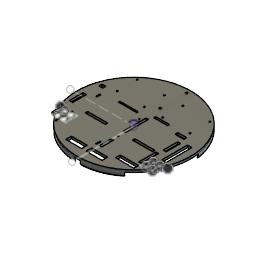
base (Autodesk Fusion 360 design; units mm, degrees)
part number: 2026-05-09-09-08-22-540
Autodesk Fusion 360 part; units mm, degrees
note: some values were not read from the file. Chosen so that the rebuilt part matches the saved one: which face or edge a step refers to. Set by a fixed rule: which sketch regions a step uses.
(part 1 of 2)
sketch "Sketch1" plane through (0, 0, 0) normal (0, 1, 0) x (1, 0, 0)
  circle A0 centre (0, 0) radius 125
  dimension "d1" = 250
  constraint coincident A0.centre origin
  measures "d1" diameter of A0
extrude "Extrude1" add sketch "Sketch1" along normal blind 5 makes body 1
sketch "Sketch3" plane through (0, 0, 0) normal (0, -1, 0) x (1, 0, 0)
  circle A0 centre (0, 0) radius 125
  line L0 (10, -45) -> (-10, -45)
  line L1 (-10, -45) -> (-10, -205)
  line L2 (-10, -205) -> (10, -205)
  line L3 (10, -205) -> (10, -45)
  line L4 (10, -45) -> (-10, -205) construction
  line L5 (-10, -45) -> (10, -205) construction
  point P0 (0, -125)
  dimension "d6" = 20
  dimension "d7" = 160
  constraint horizontal L0
  constraint perpendicular L0 L1
  constraint parallel L0 L2
  constraint parallel L1 L3
  constraint coincident L4 P0
  constraint coincident L5 P0
  constraint coincident A0 P0
  measures "d6" distance of L1.end L2.end
  measures "d7" distance of L0.end L1.end
extrude "Extrude2" add sketch "Sketch3" along normal blind 14 contours A0 L0 L1 L3 picked at (1.1122, -71.6518) bodies 1
sketch "Sketch4" plane through (0, -14, 0) normal (0, -1, 0) x (1, 0, 0)
  arc A0 (-10, -124.5994) -> (10, -124.5994) centre (0, 0) ccw
  line L0 (10, -124.5994) -> (10, -45)
  line L1 (10, -45) -> (-10, -45)
  line L2 (-10, -45) -> (-10, -124.5994)
  circle A1 centre (0, -116) radius 2.45
  circle A2 centre (0, -58) radius 2.45
  dimension "d10" = 4.9
  dimension "d11" = 4.9
  dimension "d13" = 58
  measures "d10" diameter of A1
  measures "d11" diameter of A2
  measures "d13" vertical distance of A1.centre A2.centre
extrude "Extrude3" cut sketch "Sketch4" against normal blind 19 contours A1 | A2 bodies 1
sketch "Sketch5" plane through (0, 0, 0) normal (0, -1, 0) x (1, 0, 0)
  line L0 (10, -45) -> (10, -124.5994)
  arc A0 (10, -124.5994) -> (-10, -124.5994) centre (0, 0) ccw
  line L1 (-10, -124.5994) -> (-10, -45)
  line L2 (-10, -45) -> (10, -45)
  line L3 (90.95, 48) -> (104.95, 48)
  line L4 (104.95, 48) -> (104.95, 64)
  line L5 (104.95, 64) -> (90.95, 64)
  line L6 (90.95, 64) -> (90.95, 48)
  line L7 (112.5, 43.0811) -> (82.5, 43.0811)
  line L8 (82.5, 43.0811) -> (82.5, 68.0811)
  line L9 (82.5, 68.0811) -> (112.5, 68.0811)
  line L10 (112.5, 68.0811) -> (112.5, 43.0811)
  circle A1 centre (104.95, 64) radius 1.5
  circle A2 centre (90.95, 64) radius 1.5
  circle A3 centre (90.95, 48) radius 1.5
  circle A4 centre (104.95, 48) radius 1.5
  line L11 (0, 0) -> (0, 135.933)
  circle A5 centre (-104.95, 64) radius 1.5
  line L12 (-90.95, 64) -> (-90.95, 48)
  line L13 (-104.95, 48) -> (-104.95, 64)
  circle A6 centre (-90.95, 64) radius 1.5
  circle A7 centre (-104.95, 48) radius 1.5
  line L14 (-112.5, 43.0811) -> (-82.5, 43.0811)
  line L15 (-104.95, 64) -> (-90.95, 64)
  line L16 (-112.5, 68.0811) -> (-112.5, 43.0811)
  line L17 (-90.95, 48) -> (-104.95, 48)
  line L18 (-82.5, 43.0811) -> (-82.5, 68.0811)
  circle A8 centre (-90.95, 48) radius 1.5
  line L19 (-82.5, 68.0811) -> (-112.5, 68.0811)
  line L20 (-112.5, 43.0811) -> (-117.3415, 43.0811)
  line L21 (112.5, 43.0811) -> (117.3415, 43.0811)
  line L22 (-82.5, 55.5811) -> (-112.5, 55.5811) construction
  line L23 (-97.5, 43.0811) -> (-97.5, 55.5811) construction
  line L24 (0, 0) -> (-140, 0) construction
  dimension "d22" = 14
  dimension "d23" = 16
  dimension "d24" = 93
  dimension "d29" = 30
  dimension "d30" = 25
  dimension "d32" = 7.55
  dimension "d33" = 4.0811
  dimension "d34" = 3
  dimension "d35" = 3
  dimension "d36" = 3
  dimension "d37" = 3
  dimension "d145" = 225
  constraint horizontal L3
  constraint vertical L4
  constraint horizontal L5
  constraint vertical L6
  constraint horizontal L7
  constraint vertical L8
  constraint horizontal L9
  constraint vertical L10
  constraint coincident L4.end L5.start
  constraint coincident L5.end L6.start
  constraint coincident L3.start L6.end
  constraint coincident L3.end L4.start
  constraint coincident A0.centre L11.start
  constraint vertical L11
  constraint symmetric L3.start L11 L12.end
  constraint symmetric L3.end L11 L13.start
  constraint symmetric L4.end L11 A5.centre
  constraint symmetric L5.end L11 L12.start
  constraint symmetric L7.start L11 L14.start
  constraint symmetric L7.end L11 L14.end
  constraint symmetric L8.end L11 L18.end
  constraint symmetric L9.end L11 L16.start
  constraint symmetric A1 L11 A5
  constraint symmetric A2 L11 A6
  constraint symmetric A3 L11 A8
  constraint symmetric A4 L11 A7
  constraint coincident A0 L20.end
  constraint perpendicular L16 L20
  constraint coincident A0 L21.end
  constraint perpendicular L10 L21
  constraint midpoint L18 L22.start
  constraint midpoint L16 L22.end
  constraint midpoint L14 L23.start
  constraint midpoint L22 L23.end
  constraint perpendicular L11 L24
  measures "d22" distance of L3.start L3.end
  measures "d23" distance of L3.start L5.end
  measures "d24" distance of L2 L3
  measures "d29" distance of L7.start L7.end
  measures "d30" distance of L7.start L9.end
  measures "d32" distance of L4 L10
  measures "d33" distance of L5 L9
  measures "d34" diameter of A1
  measures "d35" diameter of A2
  measures "d36" diameter of A3
  measures "d37" diameter of A4
  measures "d145" distance of L10 L16
extrude "Extrude4" add sketch "Sketch5" against normal blind 5 contours A0 L9 L10 | A0 L16 L19 bodies 1
extrude "Extrude5" cut sketch "Sketch5" against normal blind 5 contours L3 L6 A3 | L3 L6 A3 | L3 L4 A4 | L3 L4 A4 | L5 L6 A2 | L5 L6 A2 | L4 L5 A1 | L4 L5 A1 | A5 L13 L15 | A5 L13 L15 | L12 A6 L15 | L12 A6 L15 | L13 A7 L17 | L13 A7 L17 | L12 L17 A8 | L12 L17 A8 bodies 1
sketch "Sketch6" plane through (0, 5, 0) normal (0, 1, 0) x (-1, 0, 0)
  line L0 (112.5, 54.4862) -> (112.5, 68.0811)
  line L1 (112.5, 68.0811) -> (104.833, 68.0811)
  arc A0 (104.833, 68.0811) -> (-104.833, 68.0811) centre (0, 0) ccw
  line L2 (-104.833, 68.0811) -> (-112.5, 68.0811)
  line L3 (-112.5, 68.0811) -> (-112.5, 54.4862)
  circle A1 centre (0, -58) radius 2.45
  circle A2 centre (0, -116) radius 2.45
  circle A3 centre (104.95, 48) radius 1.5
  circle A4 centre (90.95, 64) radius 1.5
  circle A5 centre (90.95, 48) radius 1.5
  circle A6 centre (-90.95, 64) radius 1.5
  circle A7 centre (-90.95, 48) radius 1.5
  circle A8 centre (-104.95, 48) radius 1.5
  circle A9 centre (0, -58) radius 5
  circle A10 centre (0, -116) radius 5
  line L4 (-97.9276, 40.2238) -> (-97.9276, 63.5811)
  circle A11 centre (-105.0292, 44.701) radius 1.5
  circle A12 centre (-90.9905, 60.7002) radius 1.5
  circle A13 centre (-90.8662, 44.7011) radius 1.5
  circle A14 centre (-104.8647, 60.7002) radius 1.5
  circle A15 centre (-104.989, 44.7011) radius 1.5
  line L5 (0, 0) -> (0, 94)
  circle A16 centre (105.0292, 44.701) radius 1.5
  circle A17 centre (90.8662, 44.7011) radius 1.5
  circle A18 centre (104.8647, 60.7002) radius 1.5
  circle A19 centre (90.8944, 60.7176) radius 1.5
  arc A20 (-112.5, 54.4862) -> (112.5, 54.4862) centre (0, 0) ccw
  circle A21 centre (104.95, 64) radius 1.5
  circle A22 centre (-104.95, 64) radius 1.5
  circle A23 centre (90.9999, 67.3221) radius 1.5
  point P0 (-104.95, 48)
  point P1 (-115.3176, 44.7)
  point P2 (-104.95, 64)
  point P3 (-90.95, 48)
  point P4 (-90.95, 64)
  dimension "d42" = 10
  dimension "d45" = 3
  dimension "d46" = 3.3
  dimension "d49" = 3
  dimension "d50" = 3
  dimension "d51" = 3.3
  dimension "d52" = 3.3
  constraint concentric A1 A9
  constraint concentric A2 A10
  constraint vertical L4
  constraint symmetric L4 A12 A14
  constraint symmetric L4 A13 A15
  constraint coincident A0.centre L5.start
  constraint vertical L5
  constraint symmetric A11 L5 A16
  constraint symmetric A13 L5 A17
  constraint symmetric A14 L5 A18
  measures "d42" diameter of A9
  measures "d45" diameter of A11
  measures "d46" distance of A11.centre P0
  measures "d49" diameter of A12
  measures "d50" diameter of A13
  measures "d51" distance of A13.centre P3
  measures "d52" distance of A12.centre P4
extrude "Extrude7" cut sketch "Sketch6" against normal blind 5 contours A11 A15 | A11 A15 | A12 | A13 | A14 | A16 | A17 | A18 | A19 | A21 | A23 bodies 1
sketch "Sketch7" plane through (0, 0, 0) normal (0, -1, 0) x (1, 0, 0)
  circle A0 centre (104.95, 48) radius 1.5
  arc A1 (10, -124.5994) -> (112.5, 54.4862) centre (0, 0) ccw
  line L0 (-10, -124.5994) -> (-10, -45)
  line L1 (-10, -45) -> (10, -45)
  line L2 (10, -45) -> (10, -124.5994)
  line L3 (112.5, 54.4862) -> (112.5, 68.0811)
  line L4 (112.5, 68.0811) -> (104.833, 68.0811)
  arc A2 (104.833, 68.0811) -> (-104.833, 68.0811) centre (0, 0) ccw
  line L5 (-104.833, 68.0811) -> (-112.5, 68.0811)
  line L6 (-112.5, 68.0811) -> (-112.5, 54.4862)
  circle A3 centre (-90.95, 64) radius 1.5
  circle A4 centre (-90.95, 48) radius 1.5
  circle A5 centre (90.95, 64) radius 1.5
  circle A6 centre (90.95, 48) radius 1.5
  circle A7 centre (-104.95, 48) radius 1.5
  line L7 (0.0614, -38.5696) -> (0.0614, 91.4304)
  line L8 (-72.4386, -5) -> (-69.4386, -5)
  line L9 (-69.4386, -5) -> (-69.4386, -10)
  line L10 (-69.4386, -10) -> (-72.4386, -10)
  line L11 (-72.4386, -10) -> (-72.4386, -5)
  line L12 (72.5614, -5) -> (69.5614, -5)
  line L13 (72.5614, -10) -> (72.5614, -5)
  line L14 (69.5614, -10) -> (72.5614, -10)
  line L15 (69.5614, -5) -> (69.5614, -10)
  line L16 (30, 28) -> (-30, 28)
  line L17 (-30, 28) -> (-30, 25)
  line L18 (-30, 25) -> (30, 25)
  line L19 (30, 25) -> (30, 28)
  arc A8 (-112.5, 54.4862) -> (-10, -124.5994) centre (0, 0) ccw
  circle A9 centre (104.95, 64) radius 1.5
  circle A10 centre (-104.95, 64) radius 1.5
  circle A11 centre (-90.9999, 67.3221) radius 1.5
  circle A12 centre (-105, 52) radius 1.5
  arc A13 (105.0133, 46.2009) -> (105.0048, 43.2011) centre (104.989, 44.7011) ccw
  arc A14 (105.0048, 43.2011) -> (105.0133, 46.2009) centre (105.0292, 44.701) ccw
  circle A15 centre (90.8662, 44.7011) radius 1.5
  circle A16 centre (-90.8944, 60.7176) radius 1.5
  circle A17 centre (-105.0292, 44.701) radius 1.5
  circle A18 centre (-104.8647, 60.7002) radius 1.5
  circle A19 centre (-90.8662, 44.7011) radius 1.5
  circle A20 centre (104.8647, 60.7002) radius 1.5
  circle A21 centre (90.9905, 60.7002) radius 1.5
  dimension "d55" = 5
  dimension "d56" = 3
  dimension "d57" = 139
  dimension "d58" = 35
  dimension "d59" = 60
  dimension "d60" = 3
  dimension "d61" = 70
  constraint vertical L7
  constraint horizontal L8
  constraint vertical L9
  constraint horizontal L10
  constraint vertical L11
  constraint symmetric L7 L8.start L12.start
  constraint symmetric L7 L8.end L12.end
  constraint symmetric L7 L9.end L14.start
  constraint symmetric L7 L10.end L13.start
  constraint horizontal L16
  constraint vertical L17
  constraint horizontal L18
  constraint vertical L19
  measures "d55" distance of L8.start L10.end
  measures "d56" distance of L9.end L10.end
  measures "d58" distance of L1 L10
  measures "d59" distance of L16.start L16.end
  measures "d60" distance of L16.start L18.end
  measures "d61" distance of L1 L18
sketch "Sketch8" plane through (0, -14, 0) normal (0, -1, 0) x (1, 0, 0)
  circle A0 centre (0, -116) radius 2.45
  circle A1 centre (0, -58) radius 2.45
  arc A2 (-10, -124.5994) -> (10, -124.5994) centre (0, 0) ccw
  line L0 (10, -124.5994) -> (10, -45)
  line L1 (10, -45) -> (-10, -45)
  line L2 (-10, -45) -> (-10, -124.5994)
  line L3 (10, -51.6115) -> (-10, -51.6115)
  line L4 (-10, -51.6115) -> (-10, -45)
  line L5 (-10, -45) -> (10, -45)
  line L6 (10, -45) -> (10, -51.6115)
  constraint horizontal L3
  constraint vertical L4
  constraint horizontal L5
  constraint vertical L6
  constraint coincident L0 L3.start
  constraint coincident L1.end L2.start
sketch "Sketch10" plane through (0, 0, 0) normal (0, -1, 0) x (1, 0, 0)
  circle A0 centre (104.95, 48) radius 1.5
  arc A1 (10, -124.5994) -> (112.5, 54.4862) centre (0, 0) ccw
  line L0 (-10, -124.5994) -> (-10, -45)
  line L1 (-10, -45) -> (10, -45)
  line L2 (10, -45) -> (10, -124.5994)
  line L3 (112.5, 54.4862) -> (112.5, 68.0811)
  line L4 (112.5, 68.0811) -> (104.833, 68.0811)
  arc A2 (104.833, 68.0811) -> (-104.833, 68.0811) centre (0, 0) ccw
  line L5 (-104.833, 68.0811) -> (-112.5, 68.0811)
  line L6 (-112.5, 68.0811) -> (-112.5, 54.4862)
  circle A3 centre (-90.95, 64) radius 1.5
  circle A4 centre (-90.95, 48) radius 1.5
  circle A5 centre (90.95, 64) radius 1.5
  circle A6 centre (90.95, 48) radius 1.5
  circle A7 centre (-104.95, 48) radius 1.5
  line L7 (10, -45) -> (54, -45)
  line L8 (54, -45) -> (54, -51.8442)
  line L9 (54, -51.8442) -> (10, -51.8442)
  line L10 (10, -51.8442) -> (10, -45)
  line L11 (-10, -45) -> (-54, -45)
  line L12 (-54, -45) -> (-54, -51.8416)
  line L13 (-54, -51.8416) -> (-10, -51.8416)
  line L14 (-10, -51.8416) -> (-10, -45)
  line L15 (30, 28) -> (74, 28)
  line L16 (74, 28) -> (74, 33)
  line L17 (74, 33) -> (30, 33)
  line L18 (30, 33) -> (30, 28)
  line L19 (-30, 28) -> (-74, 28)
  line L20 (-74, 28) -> (-74, 33)
  line L21 (-74, 33) -> (-30, 33)
  line L22 (-30, 33) -> (-30, 28)
  circle A8 centre (104.95, 64) radius 1.5
  circle A9 centre (-104.95, 64) radius 1.5
  circle A10 centre (-90.9999, 67.3221) radius 1.5
  arc A11 (105.0133, 46.2009) -> (105.0048, 43.2011) centre (104.989, 44.7011) ccw
  arc A12 (105.0048, 43.2011) -> (105.0133, 46.2009) centre (105.0292, 44.701) ccw
  circle A13 centre (90.8662, 44.7011) radius 1.5
  arc A14 (-112.5, 54.4862) -> (-10, -124.5994) centre (0, 0) ccw
  circle A15 centre (-90.8944, 60.7176) radius 1.5
  circle A16 centre (-105.0292, 44.701) radius 1.5
  circle A17 centre (-104.8647, 60.7002) radius 1.5
  circle A18 centre (-90.8662, 44.7011) radius 1.5
  circle A19 centre (104.8647, 60.7002) radius 1.5
  circle A20 centre (90.9905, 60.7002) radius 1.5
  dimension "d70" = 44
  dimension "d71" = 44
  dimension "d74" = 44
  dimension "d75" = 5
  dimension "d76" = 44
  dimension "d77" = 5
  constraint horizontal L7
  constraint vertical L8
  constraint horizontal L9
  constraint vertical L10
  constraint coincident L1.end L2.start
  constraint horizontal L11
  constraint vertical L12
  constraint horizontal L13
  constraint vertical L14
  constraint coincident L0.end L1.start
  constraint horizontal L15
  constraint vertical L16
  constraint horizontal L17
  constraint vertical L18
  constraint horizontal L19
  constraint vertical L20
  constraint horizontal L21
  constraint vertical L22
  measures "d70" distance of L12.end L13.end
  measures "d71" distance of L8.end L9.end
  measures "d74" distance of L15.start L15.end
  measures "d75" distance of L15.start L17.end
  measures "d76" distance of L19.start L19.end
  measures "d77" distance of L19.start L21.end
extrude "Extrude12" cut sketch "Sketch10" against normal blind 5 contours L15 L16 L17 L18 | L19 L20 L21 L22 bodies 1
sketch "Sketch11" plane through (0, 5, 0) normal (0, 1, 0) x (-1, 0, 0)
  line L0 (-30, 28) -> (-74, 28)
  line L1 (-74, 28) -> (-74, 33)
  line L2 (-74, 33) -> (-30, 33)
  line L3 (-30, 33) -> (-30, 28)
  line L4 (74, 33) -> (74, 28)
  line L5 (74, 28) -> (30, 28)
  line L6 (30, 28) -> (30, 33)
  line L7 (30, 33) -> (74, 33)
  line L8 (112.5, 54.4862) -> (112.5, 68.0811)
  line L9 (112.5, 68.0811) -> (104.833, 68.0811)
  arc A0 (104.833, 68.0811) -> (-104.833, 68.0811) centre (0, 0) ccw
  line L10 (-104.833, 68.0811) -> (-112.5, 68.0811)
  line L11 (-112.5, 68.0811) -> (-112.5, 54.4862)
  circle A1 centre (104.95, 48) radius 1.5
  circle A2 centre (90.95, 64) radius 1.5
  circle A3 centre (90.95, 48) radius 1.5
  circle A4 centre (-90.95, 64) radius 1.5
  circle A5 centre (-90.95, 48) radius 1.5
  circle A6 centre (-104.95, 48) radius 1.5
  line L12 (2.5, 75.7) -> (92.5, 75.7)
  line L13 (92.5, 75.7) -> (92.5, -14.3)
  line L14 (92.5, -14.3) -> (2.5, -14.3)
  line L15 (2.5, -14.3) -> (2.5, 75.7)
  circle A7 centre (92.5, 75.7) radius 1.6
  circle A8 centre (2.5, 75.7) radius 1.6
  circle A9 centre (2.5, -14.3) radius 1.6
  circle A10 centre (92.5, -14.3) radius 1.6
  circle A11 centre (92.5, -10.9) radius 1.6
  circle A12 centre (92.5, -17.7) radius 1.6
  circle A13 centre (92.5, 72.3) radius 1.6
  circle A14 centre (2.5, 72.3) radius 1.6
  arc A15 (-112.5, 54.4862) -> (112.5, 54.4862) centre (0, 0) ccw
  circle A16 centre (-104.95, 64) radius 1.5
  circle A17 centre (-104.8647, 60.7002) radius 1.5
  circle A18 centre (-90.9905, 60.7002) radius 1.5
  circle A19 centre (104.95, 64) radius 1.5
  circle A20 centre (90.9999, 67.3221) radius 1.5
  arc A21 (-105.0048, 43.2011) -> (-105.0133, 46.2009) centre (-104.989, 44.7011) ccw
  arc A22 (-105.0133, 46.2009) -> (-105.0048, 43.2011) centre (-105.0292, 44.701) ccw
  circle A23 centre (-90.8662, 44.7011) radius 1.5
  circle A24 centre (91.5428, 79.2656) radius 1.6
  circle A25 centre (2.5, 79.1) radius 1.6
  circle A26 centre (0, -116) radius 2.45
  circle A27 centre (0, -58) radius 2.45
  circle A28 centre (90.8944, 60.7176) radius 1.5
  circle A29 centre (105.0292, 44.701) radius 1.5
  circle A30 centre (104.8647, 60.7002) radius 1.5
  circle A31 centre (90.8662, 44.7011) radius 1.5
  point P0 (92.5, 75.6585)
  dimension "d78" = 90
  dimension "d79" = 90
  dimension "d80" = 20
  dimension "d81" = 3.2
  dimension "d82" = 3.2
  dimension "d83" = 3.2
  dimension "d84" = 3.2
  dimension "d85" = 3.2
  dimension "d86" = 3.2
  dimension "d87" = 3.2
  dimension "d88" = 3.2
  dimension "d89" = 3.4
  dimension "d90" = 3.4
  dimension "d91" = 3.4
  dimension "d92" = 3.4
  dimension "d148" = 3.2
  constraint horizontal L12
  constraint vertical L13
  constraint horizontal L14
  constraint vertical L15
  constraint coincident L12.end L13.start
  constraint coincident L12.start L15.end
  constraint coincident L14.end L15.start
  constraint coincident L13.end L14.start
  constraint coincident L13 A11.centre
  constraint coincident L13 A12.centre
  constraint coincident L13 A13.centre
  constraint coincident L15 A14.centre
  constraint symmetric L12 A14 A25
  measures "d78" distance of L12.start L12.end
  measures "d79" distance of L12.start L14.end
  measures "d80" distance of L8 L13
  measures "d81" diameter of A7
  measures "d82" diameter of A8
  measures "d83" diameter of A9
  measures "d84" diameter of A10
  measures "d85" diameter of A11
  measures "d86" diameter of A12
  measures "d87" diameter of A13
  measures "d88" diameter of A14
  measures "d89" distance of L12.start A14.centre
  measures "d90" distance of L12.end A13.centre
  measures "d91" distance of L13.end A11.centre
  measures "d92" distance of L13.end A12.centre
  measures "d148" diameter of A24
extrude "Extrude13" cut sketch "Sketch11" against normal blind 5 contours L12 L15 A8 | L12 L15 A8 | L12 L13 A7 | L12 L13 A7 | L15 A14 | L15 A14 | L13 A13 | L13 A13 | L14 L15 A9 | L14 L15 A9 | L13 L14 A10 | L13 L14 A10 | L13 A11 | L13 A11 | A12 bodies 1
sketch "Sketch12" plane through (0, 5, 0) normal (0, 1, 0) x (-1, 0, 0)
  circle A0 centre (92.5, -14.3) radius 1.6
  circle A1 centre (2.5, 75.7) radius 1.6
  circle A2 centre (92.5, 75.7) radius 1.6
  circle A3 centre (92.5, -17.7) radius 1.6
  circle A4 centre (92.5, -10.9) radius 1.6
  circle A5 centre (2.5, 72.3) radius 1.6
  circle A6 centre (92.5, 72.3) radius 1.6
  circle A7 centre (2.5, -14.3) radius 1.6
  line L0 (-30, 28) -> (-74, 28)
  line L1 (-74, 28) -> (-74, 33)
  line L2 (-74, 33) -> (-30, 33)
  line L3 (-30, 33) -> (-30, 28)
  line L4 (74, 33) -> (74, 28)
  line L5 (74, 28) -> (30, 28)
  line L6 (30, 28) -> (30, 33)
  line L7 (30, 33) -> (74, 33)
  line L8 (112.5, 54.4862) -> (112.5, 68.0811)
  line L9 (112.5, 68.0811) -> (104.833, 68.0811)
  arc A8 (104.833, 68.0811) -> (-104.833, 68.0811) centre (0, 0) ccw
  line L10 (-104.833, 68.0811) -> (-112.5, 68.0811)
  line L11 (-112.5, 68.0811) -> (-112.5, 54.4862)
  circle A9 centre (104.95, 48) radius 1.5
  circle A10 centre (90.95, 64) radius 1.5
  circle A11 centre (90.95, 48) radius 1.5
  circle A12 centre (-90.95, 64) radius 1.5
  circle A13 centre (-90.95, 48) radius 1.5
  circle A14 centre (-104.95, 48) radius 1.5
  line L12 (-75.5, 68.844) -> (-10.5, 68.844)
  line L13 (-10.5, 68.844) -> (-10.5, -27.156)
  line L14 (-10.5, -27.156) -> (-75.5, -27.156)
  line L15 (-75.5, -27.156) -> (-75.5, 68.844)
  circle A15 centre (-97.7344, 53.0689) radius 5.2675
  line L16 (0, 0) -> (0, 130)
  circle A16 centre (97.7344, 53.0689) radius 5.2675
  line L17 (-9.1198, 80) -> (-4.2145, 80)
  line L18 (-4.2145, 80) -> (-4.2145, 53.7294)
  line L19 (-4.2145, 53.7294) -> (-9.1198, 53.7294)
  line L20 (-9.1198, 53.7294) -> (-9.1198, 80)
  line L21 (-109.4869, 38.7801) -> (-100, 38.7801)
  line L22 (-100, 38.7801) -> (-100, -17.7685)
  line L23 (-100, -17.7685) -> (-109.4869, -17.7685)
  line L24 (-109.4869, -17.7685) -> (-109.4869, 38.7801)
  line L25 (-85, 85) -> (-45, 85)
  line L26 (-45, 85) -> (-45, 75)
  line L27 (-45, 75) -> (-85, 75)
  line L28 (-85, 75) -> (-85, 85)
  line L29 (-35, 105) -> (0, 105)
  line L30 (0, 105) -> (0, 92.7786)
  line L31 (0, 92.7786) -> (-35, 92.7786)
  line L32 (-35, 92.7786) -> (-35, 105)
  line L33 (10, 105) -> (44.7011, 105)
  line L34 (44.7011, 105) -> (44.7011, 92.7786)
  line L35 (44.7011, 92.7786) -> (10, 92.7786)
  line L36 (10, 92.7786) -> (10, 105)
  line L37 (-84.4638, 67.7606) -> (-78.4638, 67.7606)
  line L38 (-78.4638, 67.7606) -> (-78.4638, 30)
  line L39 (-78.4638, 30) -> (-84.4638, 30)
  line L40 (-84.4638, 30) -> (-84.4638, 67.7606)
  line L41 (-8.0295, 25.8787) -> (-2.8969, 25.8787)
  line L42 (-2.8969, 25.8787) -> (-2.8969, -24.0249)
  line L43 (-2.8969, -24.0249) -> (-8.0295, -24.0249)
  line L44 (-8.0295, -24.0249) -> (-8.0295, 25.8787)
  line L45 (-89.1235, 18.0619) -> (-82.9645, 18.0619)
  line L46 (-82.9645, 18.0619) -> (-82.9645, -13.0755)
  line L47 (-82.9645, -13.0755) -> (-89.1235, -13.0755)
  line L48 (-89.1235, -13.0755) -> (-89.1235, 18.0619)
  line L49 (-117.6869, -42.1284) -> (117.6869, -42.1284)
  arc A17 (-115.0015, -42.1284) -> (114.9772, -42.1284) centre (-0.0122, -0.814) ccw
  line L50 (4.8653, -42.1284) -> (111.734, -42.1284)
  line L51 (111.734, -42.1284) -> (111.734, -30)
  line L52 (111.734, -30) -> (4.8653, -30)
  line L53 (4.8653, -30) -> (4.8653, -42.1284)
  arc A18 (-112.5, 54.4862) -> (112.5, 54.4862) centre (0, 0) ccw
  circle A19 centre (-104.95, 64) radius 1.5
  circle A20 centre (-104.8647, 60.7002) radius 1.5
  circle A21 centre (-90.9905, 60.7002) radius 1.5
  circle A22 centre (104.95, 64) radius 1.5
  circle A23 centre (90.9999, 67.3221) radius 1.5
  arc A24 (-105.0048, 43.2011) -> (-105.0133, 46.2009) centre (-104.989, 44.7011) ccw
  arc A25 (-105.0133, 46.2009) -> (-105.0048, 43.2011) centre (-105.0292, 44.701) ccw
  circle A26 centre (-90.8662, 44.7011) radius 1.5
  circle A27 centre (0, -116) radius 2.45
  circle A28 centre (0, -58) radius 2.45
  circle A29 centre (90.8944, 60.7176) radius 1.5
  circle A30 centre (105.0292, 44.701) radius 1.5
  circle A31 centre (104.8647, 60.7002) radius 1.5
  circle A32 centre (90.8662, 44.7011) radius 1.5
  dimension "d95" = 65
  dimension "d96" = 96
  dimension "d97" = 37
  dimension "d104" = 6
  constraint horizontal L12
  constraint vertical L13
  constraint horizontal L14
  constraint vertical L15
  constraint coincident A8.centre L16.start
  constraint perpendicular L10 L16
  constraint symmetric A15 L16 A16
  constraint horizontal L17
  constraint vertical L18
  constraint horizontal L19
  constraint vertical L20
  constraint horizontal L21
  constraint vertical L22
  constraint horizontal L23
  constraint vertical L24
  constraint horizontal L25
  constraint vertical L26
  constraint horizontal L27
  constraint vertical L28
  constraint horizontal L29
  constraint vertical L30
  constraint horizontal L31
  constraint vertical L32
  constraint coincident L16 L30.end
  constraint horizontal L33
  constraint vertical L34
  constraint horizontal L35
  constraint vertical L36
  constraint horizontal L37
  constraint vertical L38
  constraint horizontal L39
  constraint vertical L40
  constraint horizontal L41
  constraint vertical L42
  constraint horizontal L43
  constraint vertical L44
  constraint horizontal L45
  constraint vertical L46
  constraint horizontal L47
  constraint vertical L48
  constraint coincident L49 A17.start
  constraint coincident L49 A17.end
  constraint horizontal L50
  constraint vertical L51
  constraint horizontal L52
  constraint vertical L53
  constraint coincident L49 L50.start
  measures "d95" distance of L12.start L12.end
  measures "d96" distance of L12.start L14.end
  measures "d97" distance of L11 L15
  measures "d104" distance of L37.start L37.end
extrude "Extrude15" cut sketch "Sketch12" against normal blind 5 contours A15 | A16 bodies 1
extrude "Extrude16" cut sketch "Sketch12" against normal blind 5 contours L16 L29 L30 L31 L32 | L17 L18 L19 L20 | L21 L22 L23 L24 | L25 L26 L27 L28 | L33 L34 L35 L36 | L37 L38 L39 L40 | L41 L42 L43 L44 | L45 L46 L47 L48 bodies 1
sketch "Sketch13" plane through (0, 1, 0) normal (0, 1, 0) x (-1, 0, 0)
  circle A0 centre (0, -116) radius 5
  line L0 (-10, -45) -> (-10, -51.8442)
  line L1 (-10, -51.8442) -> (-54, -51.8442)
  line L2 (-54, -51.8442) -> (-54, -45)
  line L3 (-54, -45) -> (-10, -45)
  line L4 (54, -51.8416) -> (10, -51.8416)
  line L5 (10, -51.8416) -> (10, -45)
  line L6 (10, -45) -> (54, -45)
  line L7 (54, -45) -> (54, -51.8416)
  circle A1 centre (0, -58) radius 5
  arc A2 (-115.0015, -42.1284) -> (114.9772, -42.1284) centre (-0.0122, -0.814) ccw
  line L8 (114.9772, -42.1284) -> (111.734, -42.1284)
  line L9 (-26.6988, -106.8442) -> (-53.8253, -106.8442)
  line L10 (-53.8253, -106.8442) -> (-53.8253, -109.0802)
  line L11 (-53.8253, -109.0802) -> (-26.6988, -109.0802)
  line L12 (-26.6988, -109.0802) -> (-26.6988, -106.8442)
  circle A3 centre (-17.5884, -114.3194) radius 3.5583
  circle A4 centre (-87.5884, -53.2983) radius 4.8218
  line L13 (31.9215, -34.3832) -> (74.9215, -34.3832)
  line L14 (74.9215, -34.3832) -> (74.9215, -94.3832)
  line L15 (74.9215, -94.3832) -> (31.9215, -94.3832)
  line L16 (31.9215, -94.3832) -> (31.9215, -34.3832)
  line L17 (111.734, -42.1284) -> (111.734, -30)
  line L18 (111.734, -30) -> (4.8653, -30)
  line L19 (4.8653, -30) -> (4.8653, -42.1284)
  line L20 (4.8653, -42.1284) -> (-115.0015, -42.1284)
  circle A5 centre (31.9215, -94.3832) radius 1.5
  circle A6 centre (74.9215, -94.3832) radius 1.5
  circle A7 centre (22.5523, -58.3128) radius 5
  circle A8 centre (85, -55) radius 5
  circle A9 centre (24.263, -77.1424) radius 2.25
  circle A10 centre (80, -80) radius 2.25
  dimension "d112" = 55
  dimension "d113" = 70
  dimension "d114" = 43
  dimension "d115" = 60
  dimension "d118" = 3
  dimension "d119" = 3
  dimension "d120" = 10
  dimension "d121" = 10
  dimension "d122" = 4.5
  dimension "d123" = 4.5
  constraint horizontal L9
  constraint vertical L10
  constraint horizontal L11
  constraint vertical L12
  constraint horizontal L13
  constraint vertical L14
  constraint horizontal L15
  constraint vertical L16
  constraint coincident L15.end L16.start
  constraint coincident L14.end L15.start
  measures "d112" distance of L1 L9
  measures "d113" horizontal distance of A3.centre A4.centre
  measures "d114" distance of L13.start L13.end
  measures "d115" distance of L13.start L15.end
  measures "d118" diameter of A5
  measures "d119" diameter of A6
  measures "d120" diameter of A8
  measures "d121" diameter of A7
  measures "d122" diameter of A9
  measures "d123" diameter of A10
ref_plane "WorkPlane1" through (0, 10, 0) normal (0, 1, 0) x (0, 0, 1)
sketch "Sketch14" plane through (0, 10, 0) normal (0, 1, 0) x (1, 0, 0)
  circle A0 centre (0, 0) radius 65
  dimension "d127" = 130
  constraint coincident A0.centre origin
  measures "d127" diameter of A0
sketch "Sketch15" plane through (0, 5, 0) normal (0, 1, 0) x (-1, 0, 0)
  circle A0 centre (-104.95, 48) radius 1.5
  circle A1 centre (-90.95, 48) radius 1.5
  circle A2 centre (-90.95, 64) radius 1.5
  circle A3 centre (90.95, 48) radius 1.5
  circle A4 centre (90.95, 64) radius 1.5
  circle A5 centre (104.95, 48) radius 1.5
  line L0 (112.5, 54.4862) -> (112.5, 68.0811)
  line L1 (112.5, 68.0811) -> (104.833, 68.0811)
  arc A6 (104.833, 68.0811) -> (-104.833, 68.0811) centre (0, 0) ccw
  line L2 (-104.833, 68.0811) -> (-112.5, 68.0811)
  line L3 (-112.5, 68.0811) -> (-112.5, 54.4862)
  line L4 (74, 33) -> (74, 28)
  line L5 (74, 28) -> (30, 28)
  line L6 (30, 28) -> (30, 33)
  line L7 (30, 33) -> (74, 33)
  circle A7 centre (92.5, 72.3) radius 1.6
  circle A8 centre (92.5, -10.9) radius 1.6
  circle A9 centre (92.5, -17.7) radius 1.6
  circle A10 centre (92.5, 75.7) radius 1.6
  circle A11 centre (92.5, -14.3) radius 1.6
  line L8 (0, 105) -> (0, 92.7786)
  line L9 (0, 92.7786) -> (-35, 92.7786)
  line L10 (-35, 92.7786) -> (-35, 105)
  line L11 (-35, 105) -> (0, 105)
  line L12 (-100, 38.7801) -> (-100, -17.7685)
  line L13 (-100, -17.7685) -> (-109.4869, -17.7685)
  line L14 (-109.4869, -17.7685) -> (-109.4869, 38.7801)
  line L15 (-109.4869, 38.7801) -> (-100, 38.7801)
  line L16 (44.7011, 105) -> (44.7011, 92.7786)
  line L17 (44.7011, 92.7786) -> (10, 92.7786)
  line L18 (10, 92.7786) -> (10, 105)
  line L19 (10, 105) -> (44.7011, 105)
  line L20 (-82.9645, 18.0619) -> (-82.9645, -13.0755)
  line L21 (-82.9645, -13.0755) -> (-89.1235, -13.0755)
  line L22 (-89.1235, -13.0755) -> (-89.1235, 18.0619)
  line L23 (-89.1235, 18.0619) -> (-82.9645, 18.0619)
  line L24 (-4.2145, 80) -> (-4.2145, 53.7294)
  line L25 (-9.1198, 53.7294) -> (-9.1198, 80)
  line L26 (-9.1198, 80) -> (-4.2145, 80)
  line L27 (-45, 85) -> (-45, 75)
  line L28 (-45, 75) -> (-85, 75)
  line L29 (-85, 75) -> (-85, 85)
  line L30 (-85, 85) -> (-45, 85)
  line L31 (-78.4638, 67.7606) -> (-78.4638, 30)
  line L32 (-78.4638, 30) -> (-84.4638, 30)
  line L33 (-84.4638, 30) -> (-84.4638, 67.7606)
  line L34 (-84.4638, 67.7606) -> (-78.4638, 67.7606)
  circle A12 centre (-6.976, 41.8165) radius 1.5
  line L35 (18, -24) -> (58, -24)
  line L36 (58, -24) -> (58, -27)
  line L37 (58, -27) -> (18, -27)
  line L38 (18, -27) -> (18, -24)
  circle A13 centre (0, -47.5) radius 4
  line L39 (-40.8736, -33.1025) -> (-10.8736, -33.1025)
  line L40 (-10.8736, -33.1025) -> (-10.8736, -37.1025)
  line L41 (-10.8736, -37.1025) -> (-40.8736, -37.1025)
  line L42 (-40.8736, -37.1025) -> (-40.8736, -33.1025)
  circle A14 centre (0, -47.5) radius 2
  circle A15 centre (-97.7344, 53.0689) radius 5.2675
  circle A16 centre (97.7344, 53.0689) radius 5.2675
  arc A17 (-112.5, 54.4862) -> (112.5, 54.4862) centre (0, 0) ccw
  circle A18 centre (-104.95, 64) radius 1.5
  circle A19 centre (-104.8647, 60.7002) radius 1.5
  circle A20 centre (-90.9905, 60.7002) radius 1.5
  circle A21 centre (104.95, 64) radius 1.5
  circle A22 centre (90.9999, 67.3221) radius 1.5
  arc A23 (-105.0048, 43.2011) -> (-105.0133, 46.2009) centre (-104.989, 44.7011) ccw
  arc A24 (-105.0133, 46.2009) -> (-105.0048, 43.2011) centre (-105.0292, 44.701) ccw
  circle A25 centre (-90.8662, 44.7011) radius 1.5
  line L43 (-8.0295, -24.0249) -> (-8.0295, 25.8787)
  line L44 (-8.0295, 25.8787) -> (-2.8969, 25.8787)
  line L45 (-2.8969, 25.8787) -> (-2.8969, -24.0249)
  line L46 (-2.8969, -24.0249) -> (-8.0295, -24.0249)
  line L47 (-4.2145, 53.7294) -> (-9.1198, 53.7294)
  line L48 (-30, 28) -> (-74, 28)
  line L49 (-74, 28) -> (-74, 33)
  line L50 (-74, 33) -> (-30, 33)
  line L51 (-30, 33) -> (-30, 28)
  circle A26 centre (2.5, 75.7) radius 1.6
  circle A27 centre (2.5, 72.3) radius 1.6
  circle A28 centre (2.5, -14.3) radius 1.6
  circle A29 centre (0, -116) radius 2.45
  circle A30 centre (0, -58) radius 2.45
  circle A31 centre (90.8944, 60.7176) radius 1.5
  circle A32 centre (105.0292, 44.701) radius 1.5
  circle A33 centre (104.8647, 60.7002) radius 1.5
  circle A34 centre (90.8662, 44.7011) radius 1.5
  dimension "d128" = 3
  dimension "d131" = 40
  dimension "d132" = 3
  dimension "d133" = 8
  dimension "d138" = 30
  dimension "d139" = 4
  dimension "d142" = 4
  constraint horizontal L35
  constraint vertical L36
  constraint horizontal L37
  constraint vertical L38
  constraint horizontal L39
  constraint vertical L40
  constraint horizontal L41
  constraint vertical L42
  constraint concentric A13 A14
  measures "d128" diameter of A12
  measures "d131" distance of L35.start L35.end
  measures "d132" distance of L35.start L37.end
  measures "d133" diameter of A13
  measures "d138" distance of L39.start L39.end
  measures "d139" distance of L39.start L41.end
  measures "d142" diameter of A14
extrude "Extrude22" cut sketch "Sketch15" against normal blind 5 contours A12 bodies 1
extrude "Extrude23" cut sketch "Sketch15" against normal blind 4 contours L35 L36 L37 L38 | L39 L40 L41 L42 bodies 1
extrude "Extrude24" add sketch "Sketch15" against normal blind 4 contours A13 | A14 bodies 1
extrude "Extrude26" cut sketch "Sketch5" against normal blind 5 contours A0 L10 L21 | A0 L16 L20 bodies 1
extrude "Extrude27" cut sketch "Sketch11" against normal blind 5 contours A12 | A24 | A25 bodies 1
sketch "Sketch16" plane through (0, 5, 0) normal (0, 1, 0) x (-1, 0, 0)
  line L0 (58, -24) -> (58, -27)
  line L1 (58, -27) -> (18, -27)
  line L2 (18, -27) -> (18, -24)
  line L3 (18, -24) -> (58, -24)
  line L4 (-10.8736, -33.1025) -> (-10.8736, -37.1025)
  line L5 (-10.8736, -37.1025) -> (-40.8736, -37.1025)
  line L6 (-40.8736, -37.1025) -> (-40.8736, -33.1025)
  line L7 (-40.8736, -33.1025) -> (-10.8736, -33.1025)
  circle A0 centre (-6.976, 41.8165) radius 1.5
  line L8 (-78.4638, 67.7606) -> (-78.4638, 30)
  line L9 (-78.4638, 30) -> (-84.4638, 30)
  line L10 (-84.4638, 30) -> (-84.4638, 67.7606)
  line L11 (-84.4638, 67.7606) -> (-78.4638, 67.7606)
  line L12 (-45, 85) -> (-45, 75)
  line L13 (-45, 75) -> (-85, 75)
  line L14 (-85, 75) -> (-85, 85)
  line L15 (-85, 85) -> (-45, 85)
  line L16 (-4.2145, 80) -> (-4.2145, 53.7294)
  line L17 (-4.2145, 53.7294) -> (-9.1198, 53.7294)
  line L18 (-9.1198, 53.7294) -> (-9.1198, 80)
  line L19 (-9.1198, 80) -> (-4.2145, 80)
  line L20 (-82.9645, 18.0619) -> (-82.9645, -13.0755)
  line L21 (-82.9645, -13.0755) -> (-89.1235, -13.0755)
  line L22 (-89.1235, -13.0755) -> (-89.1235, 18.0619)
  line L23 (-89.1235, 18.0619) -> (-82.9645, 18.0619)
  line L24 (44.7011, 105) -> (44.7011, 92.7786)
  line L25 (44.7011, 92.7786) -> (10, 92.7786)
  line L26 (10, 92.7786) -> (10, 105)
  line L27 (10, 105) -> (44.7011, 105)
  line L28 (-100, 38.7801) -> (-100, -17.7685)
  line L29 (-100, -17.7685) -> (-109.4869, -17.7685)
  line L30 (-109.4869, -17.7685) -> (-109.4869, 38.7801)
  line L31 (-109.4869, 38.7801) -> (-100, 38.7801)
  line L32 (0, 105) -> (0, 92.7786)
  line L33 (0, 92.7786) -> (-35, 92.7786)
  line L34 (-35, 92.7786) -> (-35, 105)
  line L35 (-35, 105) -> (0, 105)
  line L36 (-2.8969, 25.8787) -> (-2.8969, -24.0249)
  line L37 (-2.8969, -24.0249) -> (-8.0295, -24.0249)
  line L38 (-8.0295, -24.0249) -> (-8.0295, 25.8787)
  line L39 (-8.0295, 25.8787) -> (-2.8969, 25.8787)
  circle A1 centre (-97.7344, 53.0689) radius 5.2675
  circle A2 centre (97.7344, 53.0689) radius 5.2675
  circle A3 centre (92.5, -14.3) radius 1.6
  circle A4 centre (2.5, 75.7) radius 1.6
  circle A5 centre (92.5, 75.7) radius 1.6
  circle A6 centre (92.5, -17.7) radius 1.6
  circle A7 centre (92.5, -10.9) radius 1.6
  circle A8 centre (2.5, 72.3) radius 1.6
  circle A9 centre (92.5, 72.3) radius 1.6
  circle A10 centre (2.5, -14.3) radius 1.6
  line L40 (-30, 28) -> (-74, 28)
  line L41 (-74, 28) -> (-74, 33)
  line L42 (-74, 33) -> (-30, 33)
  line L43 (-30, 33) -> (-30, 28)
  line L44 (74, 33) -> (74, 28)
  line L45 (74, 28) -> (30, 28)
  line L46 (30, 28) -> (30, 33)
  line L47 (30, 33) -> (74, 33)
  circle A11 centre (-104.95, 48) radius 1.5
  circle A12 centre (90.95, 64) radius 1.5
  circle A13 centre (90.95, 48) radius 1.5
  circle A14 centre (-104.95, 64) radius 1.5
  circle A15 centre (-90.95, 64) radius 1.5
  circle A16 centre (104.95, 48) radius 1.5
  circle A17 centre (-90.95, 48) radius 1.5
  circle A18 centre (104.95, 64) radius 1.5
  circle A19 centre (0, -116) radius 2.45
  circle A20 centre (0, -58) radius 2.45
  circle A21 centre (90.8944, 60.7176) radius 1.5
  arc A22 (-105.0048, 43.2011) -> (-105.0133, 46.2009) centre (-104.989, 44.7011) ccw
  arc A23 (-105.0133, 46.2009) -> (-105.0048, 43.2011) centre (-105.0292, 44.701) ccw
  circle A24 centre (105.0292, 44.701) radius 1.5
  circle A25 centre (-104.8647, 60.7002) radius 1.5
  circle A26 centre (90.9999, 67.3221) radius 1.5
  circle A27 centre (104.8647, 60.7002) radius 1.5
  circle A28 centre (-90.8662, 44.7011) radius 1.5
  circle A29 centre (90.8662, 44.7011) radius 1.5
  circle A30 centre (-90.9905, 60.7002) radius 1.5
  line L48 (-112.5, 43.0811) -> (-117.3415, 43.0811)
  arc A31 (-117.3415, 43.0811) -> (117.3415, 43.0811) centre (0, 0) ccw
  line L49 (117.3415, 43.0811) -> (112.5, 43.0811)
  line L50 (112.5, 43.0811) -> (112.5, 68.0811)
  line L51 (112.5, 68.0811) -> (104.833, 68.0811)
  arc A32 (104.833, 68.0811) -> (-104.833, 68.0811) centre (0, 0) ccw
  line L52 (-104.833, 68.0811) -> (-112.5, 68.0811)
  line L53 (-112.5, 68.0811) -> (-112.5, 43.0811)
  circle A33 centre (91.5428, 79.2656) radius 1.6
  circle A34 centre (2.5, 79.1) radius 1.6
  line L54 (107.5823, 27.0674) -> (114.8227, 27.0674)
  line L55 (114.8227, 27.0674) -> (114.8227, -2.7993)
  line L56 (114.8227, -2.7993) -> (107.5823, -2.7993)
  line L57 (107.5823, -2.7993) -> (107.5823, 27.0674)
  constraint horizontal L54
  constraint vertical L55
  constraint horizontal L56
  constraint vertical L57
extrude "Extrude28" cut sketch "Sketch16" against normal blind 5 contours L54 L55 L56 L57 bodies 1
sketch "Sketch17" plane through (0, 0, 0) normal (0, -1, 0) x (1, 0, 0)
  circle A0 centre (-2.5, 79.1) radius 1.6
  circle A1 centre (-91.5428, 79.2656) radius 1.6
  line L0 (117.3415, 43.0811) -> (112.5, 43.0811)
  line L1 (112.5, 43.0811) -> (112.5, 68.0811)
  line L2 (112.5, 68.0811) -> (104.833, 68.0811)
  arc A2 (104.833, 68.0811) -> (-104.833, 68.0811) centre (0, 0) ccw
  line L3 (-104.833, 68.0811) -> (-112.5, 68.0811)
  line L4 (-112.5, 68.0811) -> (-112.5, 43.0811)
  line L5 (-112.5, 43.0811) -> (-117.3415, 43.0811)
  arc A3 (-117.3415, 43.0811) -> (-10, -124.5994) centre (0, 0) ccw
  line L6 (-10, -124.5994) -> (-10, -45)
  line L7 (-10, -45) -> (10, -45)
  line L8 (10, -45) -> (10, -124.5994)
  arc A4 (10, -124.5994) -> (117.3415, 43.0811) centre (0, 0) ccw
  line L9 (74, 28) -> (30, 28)
  line L10 (30, 28) -> (30, 33)
  line L11 (30, 33) -> (74, 33)
  line L12 (74, 33) -> (74, 28)
  line L13 (-74, 28) -> (-74, 33)
  line L14 (-74, 33) -> (-30, 33)
  line L15 (-30, 33) -> (-30, 28)
  line L16 (-30, 28) -> (-74, 28)
  circle A5 centre (104.95, 48) radius 1.5
  circle A6 centre (-90.95, 64) radius 1.5
  circle A7 centre (-90.95, 48) radius 1.5
  circle A8 centre (104.95, 64) radius 1.5
  circle A9 centre (90.95, 64) radius 1.5
  circle A10 centre (-104.95, 48) radius 1.5
  circle A11 centre (90.95, 48) radius 1.5
  circle A12 centre (-104.95, 64) radius 1.5
  circle A13 centre (-90.8944, 60.7176) radius 1.5
  arc A14 (105.0133, 46.2009) -> (105.0048, 43.2011) centre (104.989, 44.7011) ccw
  arc A15 (105.0048, 43.2011) -> (105.0133, 46.2009) centre (105.0292, 44.701) ccw
  circle A16 centre (-105.0292, 44.701) radius 1.5
  circle A17 centre (-90.9999, 67.3221) radius 1.5
  circle A18 centre (-104.8647, 60.7002) radius 1.5
  circle A19 centre (90.8662, 44.7011) radius 1.5
  circle A20 centre (-90.8662, 44.7011) radius 1.5
  circle A21 centre (-2.5, -14.3) radius 1.6
  circle A22 centre (-92.5, 72.3) radius 1.6
  circle A23 centre (-2.5, 72.3) radius 1.6
  circle A24 centre (-92.5, -10.9) radius 1.6
  circle A25 centre (-92.5, -17.7) radius 1.6
  circle A26 centre (-92.5, 75.7) radius 1.6
  circle A27 centre (-2.5, 75.7) radius 1.6
  circle A28 centre (-92.5, -14.3) radius 1.6
  circle A29 centre (-97.7344, 53.0689) radius 5.2675
  circle A30 centre (97.7344, 53.0689) radius 5.2675
  line L17 (2.8969, -24.0249) -> (2.8969, 25.8787)
  line L18 (2.8969, 25.8787) -> (8.0295, 25.8787)
  line L19 (8.0295, 25.8787) -> (8.0295, -24.0249)
  line L20 (8.0295, -24.0249) -> (2.8969, -24.0249)
  line L21 (0, 92.7786) -> (0, 105)
  line L22 (0, 105) -> (35, 105)
  line L23 (35, 105) -> (35, 92.7786)
  line L24 (35, 92.7786) -> (0, 92.7786)
  line L25 (100, -17.7685) -> (100, 38.7801)
  line L26 (100, 38.7801) -> (109.4869, 38.7801)
  line L27 (109.4869, 38.7801) -> (109.4869, -17.7685)
  line L28 (109.4869, -17.7685) -> (100, -17.7685)
  line L29 (-44.7011, 92.7786) -> (-44.7011, 105)
  line L30 (-44.7011, 105) -> (-10, 105)
  line L31 (-10, 105) -> (-10, 92.7786)
  line L32 (-10, 92.7786) -> (-44.7011, 92.7786)
  line L33 (82.9645, -13.0755) -> (82.9645, 18.0619)
  line L34 (82.9645, 18.0619) -> (89.1235, 18.0619)
  line L35 (89.1235, 18.0619) -> (89.1235, -13.0755)
  line L36 (89.1235, -13.0755) -> (82.9645, -13.0755)
  line L37 (4.2145, 53.7294) -> (4.2145, 80)
  line L38 (4.2145, 80) -> (9.1198, 80)
  line L39 (9.1198, 80) -> (9.1198, 53.7294)
  line L40 (9.1198, 53.7294) -> (4.2145, 53.7294)
  line L41 (45, 75) -> (45, 85)
  line L42 (45, 85) -> (85, 85)
  line L43 (85, 85) -> (85, 75)
  line L44 (85, 75) -> (45, 75)
  line L45 (78.4638, 30) -> (78.4638, 67.7606)
  line L46 (78.4638, 67.7606) -> (84.4638, 67.7606)
  line L47 (84.4638, 67.7606) -> (84.4638, 30)
  line L48 (84.4638, 30) -> (78.4638, 30)
  circle A31 centre (6.976, 41.8165) radius 1.5
  line L49 (-114.8227, -2.7993) -> (-114.8227, 27.0674)
  line L50 (-114.8227, 27.0674) -> (-107.5823, 27.0674)
  line L51 (-107.5823, 27.0674) -> (-107.5823, -2.7993)
  line L52 (-107.5823, -2.7993) -> (-114.8227, -2.7993)
  line L53 (80.0985, -87.3755) -> (20.0985, -87.3755)
  line L54 (20.0985, -87.3755) -> (20.0985, -43.3755)
  line L55 (20.0985, -43.3755) -> (80.0985, -43.3755)
  line L56 (80.0985, -43.3755) -> (80.0985, -87.3755)
  circle A32 centre (80.0985, -87.3755) radius 1.7
  circle A33 centre (80.0985, -43.3755) radius 1.7
  circle A34 centre (20.0985, -87.3755) radius 1.7
  circle A35 centre (20.0985, -43.3755) radius 1.7
  line L57 (93.3412, -30) -> (23.3412, -30)
  line L58 (23.3412, -30) -> (23.3412, 30)
  line L59 (23.3412, 30) -> (93.3412, 30)
  line L60 (93.3412, 30) -> (93.3412, -30)
  line L61 (0, -115) -> (0, -35) construction
  circle A36 centre (-80.0985, -87.3755) radius 1.7
  circle A37 centre (-80.0985, -43.3755) radius 1.7
  circle A38 centre (-20.0985, -43.3755) radius 1.7
  circle A39 centre (-20.0985, -87.3755) radius 1.7
  circle A40 centre (104.8647, 60.7002) radius 1.5
  circle A41 centre (90.9905, 60.7002) radius 1.5
  dimension "d153" = 44
  dimension "d154" = 60
  dimension "d155" = 3.4
  dimension "d156" = 3.4
  dimension "d157" = 3.4
  dimension "d158" = 3.4
  dimension "d159" = 70
  dimension "d160" = 60
  constraint horizontal L53
  constraint vertical L54
  constraint horizontal L55
  constraint vertical L56
  constraint coincident L53.start L56.end
  constraint coincident L55.end L56.start
  constraint coincident L53.end L54.start
  constraint coincident L54.end L55.start
  constraint horizontal L57
  constraint vertical L58
  constraint horizontal L59
  constraint vertical L60
  constraint parallel L6 L61
  constraint symmetric A32 L61 A36
  constraint symmetric A33 L61 A37
  constraint symmetric A34 L61 A39
  constraint symmetric A35 L61 A38
  measures "d153" distance of L53.start L55.end
  measures "d154" distance of L53.start L53.end
  measures "d155" diameter of A32
  measures "d156" diameter of A33
  measures "d157" diameter of A34
  measures "d158" diameter of A35
  measures "d159" distance of L57.start L57.end
  measures "d160" distance of L57.start L59.end
extrude "Extrude29" cut sketch "Sketch17" against normal blind 5 contours L53 L54 A34 | L53 L54 A34 | L53 L56 A32 | L53 L56 A32 | L54 L55 A35 | L54 L55 A35 | L55 L56 A33 | L55 L56 A33 | A36 | A37 | A38 | A39 bodies 1